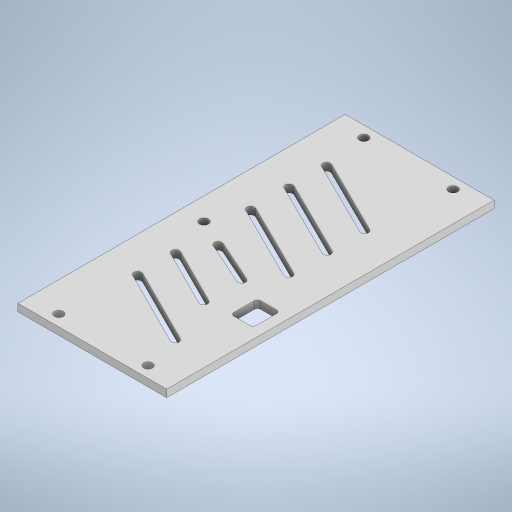
# Autodesk Inventor part: left_side
Saved by Autodesk Inventor 2024 (Build 280153000, 153)
## iProperties
Created: 2026-03-15
Part Number: left_side
Material: Generic
Document SubType Name: Modeling
Designer: HP
Density: 1 g/cm^3
Appearance: Default
Author: HP
Autodesk Inventor part; units mm, degrees
ref_plane "YZ Plane" through (0, 0, 0) normal (1, 0, 0) x (0, 1, 0)
ref_plane "XZ Plane" through (0, 0, 0) normal (0, 1, 0) x (-1, 0, 0)
ref_plane "XY Plane" through (0, 0, 0) normal (0, 0, 1) x (1, 0, 0)
sketch "Sketch1" plane through (0, 0, 0) normal (0, 1, 0) x (-1, 0, 0)
  line L0 (0, 0) -> (0, 110)
  line L1 (0, 110) -> (50, 110)
  line L2 (50, 110) -> (50, -110)
  line L3 (50, -110) -> (0, -110)
  line L4 (0, -110) -> (0, 0)
  line L5 (50, 0) -> (0, 0)
  line L6 (50, 110) -> (50, 102.5)
  line L7 (50, 102.5) -> (30, 102.5)
  line L8 (0, 110) -> (-50, 110)
  line L9 (-50, 110) -> (-50, -110)
  line L10 (-50, -110) -> (0, -110)
  circle A0 centre (30, 102.5) radius 3
  line L11 (30, 102.5) -> (-30, 102.5)
  circle A1 centre (-30, 102.5) radius 3
  circle A2 centre (30, -102.5) radius 3
  circle A3 centre (-30, -102.5) radius 3
  line L12 (30, 102.5) -> (30, -102.5)
  line L13 (-30, 102.5) -> (-30, -102.5)
  line L14 (30, 76.2) -> (-30, 50.8) construction
  line L15 (28.0508, 80.8044) -> (-31.9492, 55.4044)
  line L16 (-28.0508, 46.1956) -> (31.9492, 71.5956)
  arc A4 (31.9492, 71.5956) -> (28.0508, 80.8044) centre (30, 76.2) ccw
  arc A5 (-31.9492, 55.4044) -> (-28.0508, 46.1956) centre (-30, 50.8) ccw
  line L17 (30, 50.8) -> (-30, 25.4) construction
  line L18 (28.0508, 55.4044) -> (-31.9492, 30.0044)
  line L19 (-28.0508, 20.7956) -> (31.9492, 46.1956)
  arc A6 (31.9492, 46.1956) -> (28.0508, 55.4044) centre (30, 50.8) ccw
  arc A7 (-31.9492, 30.0044) -> (-28.0508, 20.7956) centre (-30, 25.4) ccw
  line L20 (30, 25.4) -> (-30, 0) construction
  line L21 (28.0508, 30.0044) -> (-31.9492, 4.6044)
  line L22 (-28.0508, -4.6044) -> (31.9492, 20.7956)
  arc A8 (31.9492, 20.7956) -> (28.0508, 30.0044) centre (30, 25.4) ccw
  arc A9 (-31.9492, 4.6044) -> (-28.0508, -4.6044) centre (-30, 0) ccw
  line L23 (30, 0) -> (-30, -25.4) construction
  line L24 (28.0508, 4.6044) -> (-31.9492, -20.7956)
  line L25 (-28.0508, -30.0044) -> (31.9492, -4.6044)
  arc A10 (31.9492, -4.6044) -> (28.0508, 4.6044) centre (30, 0) ccw
  arc A11 (-31.9492, -20.7956) -> (-28.0508, -30.0044) centre (-30, -25.4) ccw
  line L26 (30, -25.4) -> (-30, -50.8) construction
  line L27 (28.0508, -20.7956) -> (-31.9492, -46.1956)
  line L28 (-28.0508, -55.4044) -> (31.9492, -30.0044)
  arc A12 (31.9492, -30.0044) -> (28.0508, -20.7956) centre (30, -25.4) ccw
  arc A13 (-31.9492, -46.1956) -> (-28.0508, -55.4044) centre (-30, -50.8) ccw
  line L29 (30, -50.8) -> (-30, -76.2) construction
  line L30 (28.0508, -46.1956) -> (-31.9492, -71.5956)
  line L31 (-28.0508, -80.8044) -> (31.9492, -55.4044)
  arc A14 (31.9492, -55.4044) -> (28.0508, -46.1956) centre (30, -50.8) ccw
  arc A15 (-31.9492, -71.5956) -> (-28.0508, -80.8044) centre (-30, -76.2) ccw
  point P0 (0, 63.5)
  point P1 (0, 38.1)
  point P2 (0, 12.7)
  point P3 (0, -12.7)
  point P4 (0, -38.1)
  point P5 (0, -63.5)
  dimension "d0" = 110
  dimension "d1" = 50
  dimension "d2" = 220
  dimension "d3" = 7.5
  dimension "d4" = 20
  dimension "d5" = 50
  dimension "d6" = 6
  dimension "d7" = 60
  dimension "d8" = 6
  dimension "d9" = 10
  dimension "d10" = 10
  dimension "d11" = 10
  dimension "d12" = 10
  dimension "d13" = 10
  dimension "d14" = 10
  constraints: 76 end point, 24 point on circle, 24 tangent, 16 centre point, 11 point on line, 10 parallel, 9 midpoint, 6 perpendicular, 3 horizontal, 2 coincident, 2 symmetric about line, 1 vertical, 2 other
  measures "d0" distance of L0.start L0.end
  measures "d1" distance of L0.end L1.end
  measures "d2" distance of L1.end L2.end
  measures "d3" distance of L1.end L6.end
  measures "d4" distance of L6.end L7.end
  measures "d5" distance of L0.end L8.end
  measures "d6" diameter of A0
  measures "d7" distance of L11.start L11.end
  measures "d8" diameter of A1
  measures "d9" diameter of A5
  measures "d10" diameter of A7
  measures "d11" diameter of A9
  measures "d12" diameter of A11
  measures "d13" diameter of A13
  measures "d14" diameter of A15
extrude "Extrusion1" add sketch "Sketch1" along normal blind 5 contours L4 L24 L13 A9 L22 L0 | L5 L24 L4 | L0 L22 L12 A10 L24 L5 | L21 L13 A7 L19 L0 | L0 L19 L12 A8 L21 | L22 A8 L12 L19 A6 L16 A4 A0 L7 L2 L5 A10 | L25 L12 A12 L27 L4 | L4 L27 L13 A11 L25 | L24 A11 L13 L27 A13 L30 A15 L31 L4 L10 L9 L8 L0 L11 A1 L15 A5 L18 A7 L21 A9 | L25 A10 L5 L2 L3 L4 L31 A14 L12 L28 A12 | L18 L13 A5 L16 L0 | L0 L16 L12 A6 L18 | L28 L12 A14 L30 L4 | L4 L30 L13 A13 L28 | L7 A0 L11 L0 L1 L2 | L15 L13 A1 L11 L0 | L0 L11 A0 L12 A4 L15
sketch "Sketch2" plane through (0, 5, 0) normal (0, 1, 0) x (1, 0, 0)
  line L0 (31.9492, -55.4044) -> (-28.0508, -80.8044) projected
  line L1 (-28.0508, -80.8044) -> (31.9492, -55.4044)
  line L2 (-31.9492, -71.5956) -> (28.0508, -46.1956) projected
  line L3 (-31.9492, -71.5956) -> (28.0508, -46.1956)
  arc A0 (31.9492, -55.4044) -> (28.0508, -46.1956) centre (30, -50.8) ccw projected
  arc A1 (31.9492, -55.4044) -> (28.0508, -46.1956) centre (30, -50.8) ccw
  arc A2 (-31.9492, -71.5956) -> (-28.0508, -80.8044) centre (-30, -76.2) ccw projected
  arc A3 (-31.9492, -71.5956) -> (-28.0508, -80.8044) centre (-30, -76.2) ccw
  arc A4 (-31.9492, -46.1956) -> (-28.0508, -55.4044) centre (-30, -50.8) ccw projected
  arc A5 (-31.9492, -46.1956) -> (-28.0508, -55.4044) centre (-30, -50.8) ccw
  arc A6 (31.9492, -30.0044) -> (28.0508, -20.7956) centre (30, -25.4) ccw projected
  arc A7 (31.9492, -30.0044) -> (28.0508, -20.7956) centre (30, -25.4) ccw
  line L4 (31.9492, -30.0044) -> (-28.0508, -55.4044)
  line L5 (-31.9492, -46.1956) -> (28.0508, -20.7956)
  point P0 (0, 0)
  constraints: 8 end point, 8 point on circle, 4 centre point, 4 tangent, 3 equal length
extrude "Extrusion2" add sketch "Sketch2" against normal blind 5
sketch "Sketch3" plane through (0, 5, 0) normal (0, 1, 0) x (1, 0, 0)
  line L0 (50, -110) -> (50, 110) projected
  line L1 (-50, -110) -> (50, -110) projected
  line L2 (50, -110) -> (-50, -110)
  line L3 (50, -110) -> (25, -110)
  line L4 (25, -110) -> (25, -50)
  line L5 (25, -50) -> (17.5, -50)
  line L6 (17.5, -50) -> (17.5, -35)
  line L7 (17.5, -35) -> (32.5, -35)
  line L8 (32.5, -35) -> (32.5, -50)
  line L9 (32.5, -50) -> (25, -50)
  line L10 (-25.409, -50.782) -> (-0.009, -38.082) construction
  line L11 (-23.1729, -55.2541) -> (2.2271, -42.5541)
  line L12 (-2.2451, -33.6099) -> (-27.6451, -46.3099)
  arc A0 (-27.6451, -46.3099) -> (-23.1729, -55.2541) centre (-25.409, -50.782) ccw
  arc A1 (2.2271, -42.5541) -> (-2.2451, -33.6099) centre (-0.009, -38.082) ccw
  line L13 (-25.409, -76.2) -> (-0.009, -63.5) construction
  line L14 (-23.1729, -80.6721) -> (2.2271, -67.9721)
  line L15 (-2.2451, -59.0279) -> (-27.6451, -71.7279)
  arc A2 (-27.6451, -71.7279) -> (-23.1729, -80.6721) centre (-25.409, -76.2) ccw
  arc A3 (2.2271, -67.9721) -> (-2.2451, -59.0279) centre (-0.009, -63.5) ccw
  point P0 (0, 0)
  point P1 (-12.709, -44.432)
  point P2 (-12.709, -69.85)
  dimension "d19" = 25
  dimension "d20" = 60
  dimension "d21" = 7.5
  dimension "d22" = 15
  dimension "d23" = 15
  dimension "d24" = 10
  dimension "d25" = 10
  constraints: 32 end point, 8 point on circle, 8 tangent, 6 perpendicular, 4 centre point, 4 equal length, 2 midpoint, 2 point on line
  measures "d19" distance of L0.start L3.end
  measures "d20" distance of L3.end L4.end
  measures "d21" distance of L4.end L5.end
  measures "d22" distance of L5.end L6.end
  measures "d23" distance of L6.end L7.end
  measures "d24" diameter of A1
  measures "d25" diameter of A3
extrude "Extrusion3" cut sketch "Sketch3" against normal blind 5
fillet "Face Fillet1" radius 2 1 edges at (17.5, 2.5, 50)
fillet "Face Fillet2" radius 2 1 edges at (32.5, 2.5, 50)
fillet "Face Fillet3" radius 2 1 edges at (17.5, 2.5, 35)
fillet "Face Fillet4" radius 2 1 edges at (32.5, 2.5, 35)
sketch "Sketch4" plane through (0, 5, 0) normal (0, 1, 0) x (1, 0, 0)
  line L0 (-31.9492, 4.6044) -> (28.0508, 30.0044) projected
  line L1 (-31.9492, 4.6044) -> (28.0508, 30.0044)
  line L2 (31.9492, 20.7956) -> (-28.0508, -4.6044) projected
  line L3 (31.9492, 20.7956) -> (-28.0508, -4.6044)
  arc A0 (-31.9492, 4.6044) -> (-28.0508, -4.6044) centre (-30, 0) ccw
  arc A1 (31.9492, 20.7956) -> (28.0508, 30.0044) centre (30, 25.4) ccw projected
  arc A2 (31.9492, 20.7956) -> (28.0508, 30.0044) centre (30, 25.4) ccw
  point P0 (0, 0)
  constraints: 4 end point, 4 point on circle, 3 tangent, 2 centre point, 2 collinear
extrude "Extrusion4" add sketch "Sketch4" against normal blind 5
sketch "Sketch5" plane through (0, 5, 0) normal (0, 1, 0) x (1, 0, 0)
  line L0 (-50, 110) -> (-50, -110) projected
  line L1 (-50, -110) -> (-50, 0)
  line L2 (-50, 0) -> (-35, 0)
  circle A0 centre (-35, 0) radius 3
  line L3 (25.3921, 25.4185) -> (-19.0579, 6.3685) construction
  line L4 (23.4225, 30.0142) -> (-21.0275, 10.9642)
  line L5 (-17.0883, 1.7728) -> (27.3617, 20.8228)
  arc A1 (27.3617, 20.8228) -> (23.4225, 30.0142) centre (25.3921, 25.4185) ccw
  arc A2 (-21.0275, 10.9642) -> (-17.0883, 1.7728) centre (-19.0579, 6.3685) ccw
  point P0 (0, 0)
  point P1 (3.1671, 15.8935)
  dimension "d34" = 15
  dimension "d35" = 6
  dimension "d36" = 10
  constraints: 12 end point, 4 point on circle, 4 tangent, 3 centre point, 2 midpoint, 1 coincident, 1 horizontal, 1 parallel
  measures "d34" distance of L1.end L2.end
  measures "d35" diameter of A0
  measures "d36" diameter of A2
extrude "Extrusion5" cut sketch "Sketch5" against normal blind 5
sketch "Sketch6" plane through (0, 5, 0) normal (0, 1, 0) x (1, 0, 0)
  circle A0 centre (30, -102.5) radius 3 projected
  line L0 (30, -102.5) -> (30, -95)
  line L1 (30, -95) -> (30, -42)
  line L2 (30, -42) -> (40, -42)
  line L3 (40, -42) -> (25, -42)
  line L4 (25, -42) -> (25, -27)
  line L5 (25, -27) -> (40, -27)
  line L6 (40, -27) -> (40, -42)
  line L7 (32.5, -48) -> (32.5, -42)
  line L8 (32.5, -37) -> (32.5, -48) projected
  line L9 (19.5, -35) -> (30.5, -35) projected
  line L10 (25, -35) -> (19.5, -35)
  line L11 (30.5, -50) -> (19.5, -50)
  line L12 (17.5, -48) -> (17.5, -37)
  arc A1 (19.5, -35) -> (17.5, -37) centre (19.5, -37) ccw projected
  arc A2 (17.5, -48) -> (19.5, -50) centre (19.5, -48) ccw projected
  arc A3 (17.5, -48) -> (19.5, -50) centre (19.5, -48) ccw
  arc A4 (19.5, -35) -> (17.5, -37) centre (19.5, -37) ccw
  arc A5 (30.5, -50) -> (32.5, -48) centre (30.5, -48) ccw projected
  arc A6 (30.5, -50) -> (32.5, -48) centre (30.5, -48) ccw
  line L13 (40, -27) -> (43, -27)
  line L14 (43, -27) -> (43, -45)
  line L15 (43, -45) -> (25, -45)
  line L16 (25, -45) -> (25, -27)
  point P0 (0, 0)
  dimension "d39" = 7.5
  dimension "d40" = 53
  dimension "d41" = 10
  dimension "d42" = 15
  dimension "d43" = 15
  dimension "d50" = 3
  dimension "d51" = 18
  constraints: 30 end point, 7 point on circle, 5 perpendicular, 4 horizontal, 3 centre point, 3 tangent, 2 midpoint, 2 vertical, 1 collinear, 1 point on line
  measures "d39" distance of L0.start L0.end
  measures "d40" distance of L0.end L1.end
  measures "d41" distance of L1.end L2.end
  measures "d42" distance of L2.end L3.end
  measures "d43" distance of L3.end L4.end
  measures "d50" distance of L5.end L13.end
  measures "d51" distance of L13.end L14.end
extrude "Extrusion6" cut sketch "Sketch6" against normal blind 5 contours L3 L4 L5 L6 L2
sketch "Sketch7" plane through (0, 5, 0) normal (0, 1, 0) x (1, 0, 0)
  line L0 (32.5, -42) -> (40, -42) projected
  line L1 (40, -42) -> (25, -42)
  line L2 (40, -27) -> (25, -27) projected
  line L3 (25, -42) -> (25, -27)
  line L4 (32.5, -42) -> (32.5, -48) projected
  line L5 (32.5, -42) -> (32.5, -48)
  line L6 (19.5, -35) -> (25, -35) projected
  line L7 (25, -35) -> (19.5, -35)
  arc A0 (19.5, -35) -> (17.5, -37) centre (19.5, -37) ccw projected
  line L8 (17.5, -37) -> (17.5, -48)
  line L9 (30.5, -50) -> (19.5, -50) projected
  line L10 (19.5, -50) -> (30.5, -50)
  arc A1 (17.5, -48) -> (19.5, -50) centre (19.5, -48) ccw projected
  arc A2 (17.5, -48) -> (19.5, -50) centre (19.5, -48) ccw
  arc A3 (19.5, -35) -> (17.5, -37) centre (19.5, -37) ccw
  arc A4 (30.5, -50) -> (32.5, -48) centre (30.5, -48) ccw
  point P0 (0, 0)
  dimension "d46" = 15
  constraints: 12 end point, 7 point on circle, 3 centre point, 3 horizontal, 3 tangent, 1 collinear, 1 vertical
  measures "d46" distance of L0.end L1.end
extrude "Extrusion7" add sketch "Sketch7" against normal blind 5
fillet "Fillet1" radius 2 4 edges at (25, 2.5, 42) (25, 2.5, 27) (40, 2.5, 42) (40, 2.5, 27)
sketch "Sketch8" plane through (0, 5, 0) normal (0, 1, 0) x (1, 0, 0)
  line L0 (40, -29) -> (40, -40) projected
  line L1 (40, -34.5) -> (43, -34.5)
  line L2 (38, -27) -> (27, -27) projected
  line L3 (32.5, -27) -> (49.9944, -27)
  line L4 (43, -34.5) -> (43, -27)
  line L5 (43, -27) -> (43, -45)
  line L6 (43, -45) -> (25, -45)
  line L7 (25, -45) -> (25, -27)
  line L8 (25, -27) -> (43, -27)
  line L9 (43, -45) -> (28, -45)
  line L10 (28, -45) -> (28, -27)
  point P0 (0, 0)
  dimension "d52" = 3
  dimension "d53" = 18
  dimension "d54" = 18
  dimension "d55" = 15
  constraints: 18 end point, 4 perpendicular, 4 point on line, 2 horizontal, 2 midpoint, 1 collinear
  measures "d52" distance of L1.start L1.end
  measures "d53" distance of L4.end L5.end
  measures "d54" distance of L5.end L6.end
  measures "d55" distance of L5.end L9.end
extrude "Extrusion8" cut sketch "Sketch8" against normal blind 10 contours L3 L4 L5 L6 L10 L2
sketch "Sketch9" plane through (0, 5, 0) normal (0, 1, 0) x (1, 0, 0)
  line L0 (27, -42) -> (28, -42) projected
  line L1 (28, -42) -> (28, -27)
  line L2 (43, -27) -> (27, -27) projected
  line L3 (28, -42) -> (28, -45) projected
  line L4 (28, -42) -> (27, -42)
  line L5 (28, -27) -> (27, -27)
  line L6 (25, -29) -> (25, -40) projected
  line L7 (25, -40) -> (25, -29)
  arc A0 (25, -40) -> (27, -42) centre (27, -40) ccw projected
  arc A1 (25, -40) -> (27, -42) centre (27, -40) ccw
  arc A2 (27, -27) -> (25, -29) centre (27, -29) ccw
  point P0 (0, 0)
  constraints: 8 end point, 4 point on circle, 2 centre point, 2 vertical, 1 collinear, 1 perpendicular, 1 point on line
extrude "Extrusion9" add sketch "Sketch9" against normal blind 5
fillet "Fillet2" radius 2 4 edges at (28, 2.5, 45) (28, 2.5, 27) (43, 2.5, 45) (43, 2.5, 27)
sketch "Sketch10" plane through (0, 5, 0) normal (0, 1, 0) x (1, 0, 0)
  arc A0 (2.2271, -67.9721) -> (-2.2451, -59.0279) centre (-0.009, -63.5) ccw projected
  line L0 (-23.1729, -55.2541) -> (2.2271, -42.5541) projected
  line L1 (-23.1729, -55.2541) -> (2.2271, -42.5541)
  line L2 (-2.2451, -33.6099) -> (-27.6451, -46.3099) projected
  line L3 (-27.6451, -46.3099) -> (-2.2451, -33.6099)
  line L4 (31.9492, -4.6044) -> (-28.0508, -30.0044) projected
  line L5 (-28.0508, -30.0044) -> (31.9492, -4.6044)
  line L6 (-31.9492, -20.7956) -> (28.0508, 4.6044) projected
  line L7 (-31.9492, -20.7956) -> (28.0508, 4.6044)
  line L8 (-17.0883, 1.7728) -> (27.3617, 20.8228) projected
  line L9 (-17.0883, 1.7728) -> (27.3617, 20.8228)
  line L10 (23.4225, 30.0142) -> (-21.0275, 10.9642) projected
  line L11 (-21.0275, 10.9642) -> (23.4225, 30.0142)
  line L12 (31.9492, 46.1956) -> (-28.0508, 20.7956) projected
  line L13 (-28.0508, 20.7956) -> (31.9492, 46.1956)
  line L14 (-31.9492, 30.0044) -> (28.0508, 55.4044) projected
  line L15 (-31.9492, 30.0044) -> (28.0508, 55.4044)
  line L16 (31.9492, 71.5956) -> (-28.0508, 46.1956) projected
  line L17 (-28.0508, 46.1956) -> (31.9492, 71.5956)
  line L18 (-31.9492, 55.4044) -> (28.0508, 80.8044) projected
  line L19 (-31.9492, 55.4044) -> (28.0508, 80.8044)
  arc A1 (2.2271, -67.9721) -> (-2.2451, -59.0279) centre (-0.009, -63.5) ccw
  arc A2 (-27.6451, -46.3099) -> (-23.1729, -55.2541) centre (-25.409, -50.782) ccw
  arc A3 (2.2271, -42.5541) -> (-2.2451, -33.6099) centre (-0.009, -38.082) ccw
  arc A4 (-31.9492, -20.7956) -> (-28.0508, -30.0044) centre (-30, -25.4) ccw
  arc A5 (31.9492, -4.6044) -> (28.0508, 4.6044) centre (30, 0) ccw
  arc A6 (-21.0275, 10.9642) -> (-17.0883, 1.7728) centre (-19.0579, 6.3685) ccw
  arc A7 (-27.6451, -71.7279) -> (-23.1729, -80.6721) centre (-25.409, -76.2) ccw projected
  arc A8 (-27.6451, -71.7279) -> (-23.1729, -80.6721) centre (-25.409, -76.2) ccw
  line L20 (-23.1729, -80.6721) -> (2.2271, -67.9721) projected
  line L21 (-23.1729, -80.6721) -> (2.2271, -67.9721)
  line L22 (-27.6451, -71.7279) -> (-2.2451, -59.0279)
  arc A9 (-27.6451, -46.3099) -> (-23.1729, -55.2541) centre (-25.409, -50.782) ccw
  arc A10 (-31.9492, 30.0044) -> (-28.0508, 20.7956) centre (-30, 25.4) ccw
  arc A11 (-31.9492, 55.4044) -> (-28.0508, 46.1956) centre (-30, 50.8) ccw projected
  arc A12 (-31.9492, 55.4044) -> (-28.0508, 46.1956) centre (-30, 50.8) ccw
  arc A13 (31.9492, 71.5956) -> (28.0508, 80.8044) centre (30, 76.2) ccw
  arc A14 (27.3617, 20.8228) -> (23.4225, 30.0142) centre (25.3921, 25.4185) ccw
  arc A15 (31.9492, 46.1956) -> (28.0508, 55.4044) centre (30, 50.8) ccw
  point P0 (0, 0)
  constraints: 26 point on circle, 24 end point, 21 tangent, 13 centre point, 10 collinear, 1 concentric
extrude "Extrusion10" add sketch "Sketch10" against normal blind 5
sketch "Sketch11" plane through (0, 5, 0) normal (0, 1, 0) x (1, 0, 0)
  line L0 (-26.5539, -53.0299) -> (24.2875, -78.4785) construction
  line L1 (-27.6729, -55.2655) -> (23.1685, -80.7141)
  line L2 (25.4065, -76.2429) -> (-25.4349, -50.7944)
  arc A0 (-25.4349, -50.7944) -> (-27.6729, -55.2655) centre (-26.5539, -53.0299) ccw
  arc A1 (23.1685, -80.7141) -> (25.4065, -76.2429) centre (24.2875, -78.4785) ccw
  line L3 (-26.5539, -27.6193) -> (11.7561, -46.7953) construction
  line L4 (-27.6729, -29.8549) -> (10.6371, -49.0309)
  line L5 (12.8751, -44.5598) -> (-25.4349, -25.3837)
  arc A2 (-25.4349, -25.3837) -> (-27.6729, -29.8549) centre (-26.5539, -27.6193) ccw
  arc A3 (10.6371, -49.0309) -> (12.8751, -44.5598) centre (11.7561, -46.7953) ccw
  line L6 (-16.9103, -8.6065) -> (11.8587, -21.41) construction
  line L7 (-17.9268, -10.8906) -> (10.8422, -23.694)
  line L8 (12.8751, -19.1259) -> (-15.8938, -6.3225)
  arc A4 (-15.8938, -6.3225) -> (-17.9268, -10.8906) centre (-16.9103, -8.6065) ccw
  arc A5 (10.8422, -23.694) -> (12.8751, -19.1259) centre (11.8587, -21.41) ccw
  line L9 (-26.5433, 22.907) -> (24.2981, -2.2409) construction
  line L10 (-27.6517, 20.6662) -> (23.1897, -4.4817)
  line L11 (25.4065, 0) -> (-25.4349, 25.1479)
  arc A6 (-25.4349, 25.1479) -> (-27.6517, 20.6662) centre (-26.5433, 22.907) ccw
  arc A7 (23.1897, -4.4817) -> (25.4065, 0) centre (24.2981, -2.2409) ccw
  line L12 (-26.5433, 48.7204) -> (24.2981, 23.5725) construction
  line L13 (-27.6517, 46.4796) -> (23.1897, 21.3317)
  line L14 (25.4065, 25.8134) -> (-25.4349, 50.9613)
  arc A8 (-25.4349, 50.9613) -> (-27.6517, 46.4796) centre (-26.5433, 48.7204) ccw
  arc A9 (23.1897, 21.3317) -> (25.4065, 25.8134) centre (24.2981, 23.5725) ccw
  line L15 (-26.5433, 73.908) -> (24.2981, 48.7601) construction
  line L16 (-27.6517, 71.6672) -> (23.1897, 46.5192)
  line L17 (25.4065, 51.001) -> (-25.4349, 76.1489)
  arc A10 (-25.4349, 76.1489) -> (-27.6517, 71.6672) centre (-26.5433, 73.908) ccw
  arc A11 (23.1897, 46.5192) -> (25.4065, 51.001) centre (24.2981, 48.7601) ccw
  point P0 (0, 0)
  point P1 (-1.1332, -65.7542)
  point P2 (-7.3989, -37.2073)
  point P3 (-2.5258, -15.0082)
  point P4 (-1.1226, 10.3331)
  point P5 (-1.1226, 36.1465)
  point P6 (-1.1226, 61.3341)
  dimension "d63" = 5
  dimension "d64" = 5
  dimension "d65" = 5
  dimension "d66" = 5
  dimension "d67" = 5
  dimension "d68" = 5
  constraints: 48 end point, 24 point on circle, 24 tangent, 12 centre point, 8 parallel, 6 midpoint
  measures "d63" diameter of A1
  measures "d64" diameter of A3
  measures "d65" diameter of A5
  measures "d66" diameter of A7
  measures "d67" diameter of A9
  measures "d68" diameter of A11
extrude "Extrusion11" cut sketch "Sketch11" against normal blind 5
body "Solid1"
